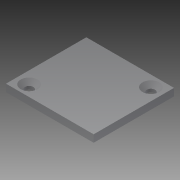
# Autodesk Inventor part: 13_1087_014
Saved by Autodesk Inventor 2014 (Build 180170000, 170)
## iProperties
Created: 2013-08-09
Part Number: 13_1087_014
Material: Allgemein
Document SubType Name: Modeling
Designer: vogel
Density: 1 g/cm^3
Appearance: Polycarbonat - klar
Author: vogel
Autodesk Inventor part; units mm, degrees
ref_plane "YZ Plane" through (0, 0, 0) normal (1, 0, 0) x (0, 1, 0)
ref_plane "XZ Plane" through (0, 0, 0) normal (0, 1, 0) x (-1, 0, 0)
ref_plane "XY Plane" through (0, 0, 0) normal (0, 0, 1) x (1, 0, 0)
sketch "Skizze1" plane through (0, 0, 0) normal (0, 0, 1) x (1, 0, 0)
  line L0 (-7.2, 0) -> (43.2, 0) projected
  line L1 (0, -6.6) -> (0, 39.6) projected
  line L2 (0, 0) -> (36, 0)
  line L3 (36, 0) -> (36, 33)
  line L4 (36, 33) -> (0, 33)
  line L5 (0, 33) -> (0, 0)
  dimension "d0" = 36
  dimension "d1" = 33
  constraints: 8 end point, 2 parallel, 1 horizontal, 1 perpendicular
  measures "d0" distance of L3.end L4.end
  measures "d1" distance of L4.end L2.start
extrude "Extrusion1" add sketch "Skizze1" along normal blind 3
sketch "Skizze2" plane through (0, 0, 3) normal (0, 0, 1) x (1, 0, 0)
  line L0 (0, 0) -> (36, 0) projected
  line L1 (36, 0) -> (36, 33) projected
  line L2 (36, 33) -> (0, 33) projected
  line L3 (0, 33) -> (0, 0) projected
  line L4 (5, 28) -> (31, 28)
  line L5 (31, 28) -> (31, 5)
  line L6 (31, 5) -> (5, 5)
  line L7 (5, 5) -> (5, 28)
  line L8 (18, 33) -> (18, 0)
  line L9 (36, 16.5) -> (0, 16.5)
  dimension "d4" = 26
  dimension "d5" = 23
  constraints: 12 end point, 4 midpoint, 2 coincident, 2 parallel, 1 horizontal, 1 perpendicular, 2 other
  measures "d4" distance of L4.start L4.end
  measures "d5" distance of L4.end L5.end
hole "Bohrung1" at (31, 28, 3) at (5, 5, 3) direction (0, 0, -1) diameter 3.4 end through all countersink diameter 6.9 countersink angle 90
